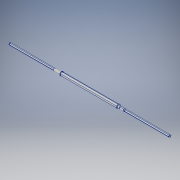
# Autodesk Inventor part: Intake Axle
Saved by Autodesk Inventor 2019.4 (Build 234330000, 330)
## iProperties
Created: 2020-01-29
Part Number: Intake Axle
Material: Aluminum 6061
Document SubType Name: Modeling
Designer: admin
Density: 2.7 g/cm^3
Appearance: Aluminum - Flat
Author: admin
Autodesk Inventor part; units mm, degrees
ref_plane "YZ Plane" through (0, 0, 0) normal (1, 0, 0) x (0, 1, 0)
ref_plane "XZ Plane" through (0, 0, 0) normal (0, 1, 0) x (-1, 0, 0)
ref_plane "XY Plane" through (0, 0, 0) normal (0, 0, 1) x (1, 0, 0)
sketch "Sketch1" plane through (0, 0, 0) normal (0, 0, 1) x (1, 0, 0)
  line L0 (0, 0) -> (0, 5)
  line L1 (221.8, 5) -> (221.8, 8)
  line L2 (221.8, 8) -> (468, 8)
  line L3 (468, 8) -> (468, 5)
  line L4 (689.8, 5) -> (689.8, 0)
  line L5 (689.8, 0) -> (0, 0)
  line L6 (468, 5) -> (474.9, 5)
  line L7 (474.9, 5) -> (474.9, 4.65)
  line L8 (474.9, 4.65) -> (476, 4.65)
  line L9 (476, 4.65) -> (476, 5)
  line L10 (476, 5) -> (492, 5)
  line L11 (492, 5) -> (492, 4.65)
  line L12 (492, 4.65) -> (493.1, 4.65)
  line L13 (493.1, 4.65) -> (493.1, 5)
  line L14 (493.1, 5) -> (689.8, 5)
  line L15 (221.8, 5) -> (0, 5)
  dimension "d2" = 246.2
  dimension "d3" = 8
  dimension "d4" = 221.8
  dimension "d5" = 221.8
  dimension "d6" = 1.1
  dimension "d7" = 1.1
  dimension "d8" = 0.35
  dimension "d11" = 5
  dimension "d12" = 5
  dimension "d13" = 8
  dimension "d14" = 16
  constraints: 32 end point, 9 perpendicular, 5 point on line, 2 horizontal, 1 vertical
  measures "d2" distance of L1.end L2.end
  measures "d3" distance between parallel lines of L5 L2
  measures "d4" distance of L0.end L1.start
  measures "d5" distance of L3.end L4.start
  measures "d6" distance of L7.end L8.end
  measures "d7" distance of L11.end L12.end
  measures "d8" distance of L6.end L7.end
  measures "d11" distance between parallel lines of L5 L15
  measures "d12" distance between parallel lines of L5 L14
  measures "d13" distance between parallel lines of L3 L9
  measures "d14" distance of L9.end L10.end
revolve "Revolution1" add sketch "Sketch1" angle 360 about axis through (689.8, 0, 0) along (-1, 0, 0)
ref_plane "Work Plane3" through (466, 0, 0) normal (1, 0, 0) x (0, 0, -1)
ref_plane "Work Plane4" through (223.8, 0, 0) normal (-1, 0, 0) x (0, 0, 1)
sketch "Sketch2" plane through (466, 0, 0) normal (1, 0, 0) x (0, 0, -1)
  circle A0 centre (0, 0) radius 8 projected
  line L0 (0, 7.1014) -> (6.15, 3.5507)
  line L1 (6.15, 3.5507) -> (6.15, -3.5507)
  line L2 (6.15, -3.5507) -> (0, -7.1014)
  line L3 (0, -7.1014) -> (-6.15, -3.5507)
  line L4 (-6.15, -3.5507) -> (-6.15, 3.5507)
  line L5 (-6.15, 3.5507) -> (0, 7.1014)
  point P0 (0, 0)
  dimension "d16" = 12.3
  constraints: 12 end point, 1 coincident, 13 other
  measures "d16" distance between parallel lines of L4 L1
extrude "Extrusion1" cut sketch "Sketch2" against normal up to surface (242.2 mm away)
sketch "Sketch3" plane through (493.1, 0, 0) normal (1, 0, 0) x (0, 0, -1)
  line L0 (-3, 4) -> (3, 4)
  circle A0 centre (0, 0) radius 5 projected
  dimension "d19" = 4
  constraints: 2 end point, 2 point on circle, 1 horizontal
  measures "d19" distance from line of A0.centre L0
extrude "Extrusion2" cut sketch "Sketch3" against normal up to surface (18.2 mm away) contours A0 L0 picked at (-0.6933, 4.1823)
sketch "Sketch4" plane through (689.8, 0, 0) normal (1, 0, 0) x (0, 0, -1)
  line L0 (4.3879, 0) -> (2.1939, -3.8)
  line L1 (2.1939, -3.8) -> (-2.1939, -3.8)
  line L2 (-2.1939, -3.8) -> (-4.3879, 0)
  line L3 (-4.3879, 0) -> (-2.1939, 3.8)
  line L4 (-2.1939, 3.8) -> (2.1939, 3.8)
  line L5 (2.1939, 3.8) -> (4.3879, 0)
  circle A0 centre (0, 0) radius 5 projected
  dimension "d22" = 7.6
  constraints: 12 end point, 1 coincident, 1 horizontal, 13 other
  measures "d22" distance between parallel lines of L4 L1
extrude "Extrusion3" cut sketch "Sketch4" against normal blind 193.1
ref_plane "Work Plane1" through (687.8, 3.8, 2.1939) normal (1, 0, 0) x (0, 0, -1)
sketch "Sketch5" plane through (687.8, 3.8, 2.1939) normal (1, 0, 0) x (0, 0, -1)
  line L0 (6.5818, -3.8) -> (4.3879, 0) projected
  line L1 (4.3879, 0) -> (0, 0) projected
  line L2 (0, 0) -> (-2.1939, -3.8) projected
  line L3 (-2.1939, -3.8) -> (0, -7.6) projected
  line L4 (0, -7.6) -> (4.3879, -7.6) projected
  line L5 (4.3879, -7.6) -> (6.5818, -3.8) projected
  circle A0 centre (2.1939, -3.8) radius 3.9
  dimension "d26" = 7.8
  constraints: 1 centre point, 1 coincident
  measures "d26" diameter of A0
extrude "Extrusion4" cut sketch "Sketch5" against normal blind 1.1 contours L5 A0 L0 | A0 L1 L0 | L5 L4 A0 | A0 L2 L1 | L4 L3 A0 | A0 L3 L2
ref_plane "Work Plane2" through (344.9, -3.5507, -6.15) normal (1, 0, 0) x (0, 0, -1)
mirror "Mirror1" about plane through (344.9, -3.5507, -6.15) normal (1, 0, 0) of "Extrusion3", "Extrusion4"
equation "\"d5\" = d4"
body "Solid1"
